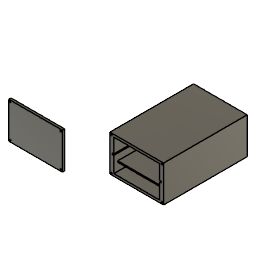
transmitter_model_v1 (Autodesk Fusion 360 design; units mm, degrees)
Autodesk Fusion 360 part; units mm, degrees
sketch "Sketch1" plane through (0, 0, 0) normal (0, 0, 1) x (1, 0, 0)
  line L0 (0, 0) -> (62, 0)
  line L1 (62, 0) -> (62, 82)
  line L2 (62, 82) -> (0, 82)
  line L3 (0, 82) -> (0, 0)
  dimension "d1" = 82
  dimension "d2" = 62
  constraint horizontal L0
  constraint vertical L1
  constraint horizontal L2
  constraint vertical L3
  constraint coincident L0.start L3.end
  measures "d1" distance of L0.start L2.end
  measures "d2" distance of L0.start L0.end
sketch "Sketch2" plane through (0, 0, 30) normal (0, 0, 1) x (-1, 0, 0)
  line L0 (0, -82) -> (0, 0)
  line L1 (0, 0) -> (-62, 0)
  line L2 (-62, 0) -> (-62, -82)
  line L3 (-62, -82) -> (0, -82)
  line L4 (-8, -8) -> (-54, -8)
  line L5 (-54, -8) -> (-54, -74)
  line L6 (-54, -74) -> (-8, -74)
  line L7 (-8, -74) -> (-8, -8)
  constraint horizontal L4
  constraint vertical L5
  constraint horizontal L6
  constraint vertical L7
sketch "Sketch3" plane through (0, 0, 0) normal (0, 0, 1) x (1, 0, 0)
  line L0 (0, 0) -> (62, 0)
  line L1 (62, 0) -> (62, 100)
  line L2 (62, 100) -> (0, 100)
  line L3 (0, 100) -> (0, 0)
  dimension "d11" = 100
  dimension "d12" = 62
  constraint horizontal L0
  constraint vertical L1
  constraint horizontal L2
  constraint vertical L3
  constraint coincident L0.start L3.end
  measures "d11" distance of L0.start L2.end
  measures "d12" distance of L0.start L0.end
extrude "Extrude3" add sketch "Sketch3" along normal blind 1.5 makes body 1
copy_body "CopyPasteBodies1" bodies 1 makes body 2
move_body "Move1" bodies 2 to x (1, 0, 0) y (0, 1, 0) z (0, 0, 1) at (-150, 0, 0)
extrude "Extrude4" add 1 faces at (62, 33.3333, 0.5) along direction (1, 0, 0) blind 8 on bodies 1 bodies 1
extrude "Extrude5" cut 1 faces at (70, 33.3333, 0.5) along direction (-1, 0, 0) blind 2 on bodies 1 bodies 1
extrude "Extrude6" add 1 faces at (45.3333, 100, 0.5) along direction (0, 1, 0) blind 6 on bodies 1 bodies 1
extrude "Extrude7" add 1 faces at (45.3333, 70.6667, 1.5) along direction (0, 0, 1) blind 44.5 on bodies 1 bodies 1
sketch "Sketch4" plane through (0, 0, 46) normal (0, 0, 1) x (-1, 0, 0)
  line L0 (-68, 0) -> (-68, -106)
  line L1 (-68, -106) -> (0, -106)
  line L2 (0, -106) -> (0, 0)
  line L3 (0, 0) -> (-68, 0)
  line L4 (0, 0) -> (-5, 0)
  line L5 (-68, 0) -> (-63, 0)
  line L6 (-5, 0) -> (-63, 0)
  line L7 (-63, 0) -> (-63, -101)
  line L8 (-63, -101) -> (-5, -101)
  line L9 (-5, -101) -> (-5, 0)
  dimension "d23" = 5
  dimension "d24" = 5
  dimension "d25" = 101
  dimension "d26" = 58
  constraint coincident L2.end L3.start
  constraint perpendicular L2 L4
  constraint coincident L0.start L3.end
  constraint perpendicular L0 L5
  constraint horizontal L6
  constraint vertical L7
  constraint horizontal L8
  constraint vertical L9
  measures "d23" distance of L2.end L4.end
  measures "d24" distance of L0.start L5.end
  measures "d25" distance of L4.end L8.end
  measures "d26" distance of L4.end L5.end
extrude "Extrude8" cut sketch "Sketch4" against normal blind 43 contours L3 L6 L7 L8 L9 bodies 1
extrude "Extrude9" add sketch "Sketch4" against normal blind 3 contours L3 L6 L7 L8 L9 bodies 1
move_body "Move2" bodies 2 to x (1, 0, 0) y (0, 1, 0) z (0, 0, 1) at (150, 0, -15)
move_body "Move3" bodies 2 to x (1, 0, 0) y (0, 1, 0) z (0, 0, 1) at (3, 0, 0)
copy_body "CopyPasteBodies2" bodies 2 makes body 3
move_body "Move4" bodies 3 to x (1, 0, 0) y (0, 1, 0) z (0, 0, 1) at (0, 0, 38)
move_body "Move5" bodies 3 to x (1, 0, 0) y (0, 1, 0) z (0, 0, 1) at (0, -100, 0)
extrude "Extrude11" add 1 faces at (23.6667, -100, 23.5) along direction (0, -1, 0) blind 3 on bodies 3 bodies 3
copy_body "CopyPasteBodies3" bodies 3 makes body 4
move_body "Move6" bodies 4 to x (1, 0, 0) y (0, 1, 0) z (0, 0, 1) at (0, 103, -10)
move_body "Move7" bodies 3 to x (1, 0, 0) y (0, 1, 0) z (0, 0, 1) at (0, 103, 0)
combine "Combine1" operation cut target body 1 tool bodies 3
combine "Combine2" operation add target body 1 tool bodies 4
sketch "Sketch5" plane through (0, 0, 0) normal (0, -1, 0) x (1, 0, 0)
  line L0 (63, 13) -> (63, 3)
  line L1 (63, 3) -> (5, 3)
  line L2 (5, 3) -> (5, 13)
  line L3 (5, 13) -> (63, 13)
  line L4 (68, 46) -> (0, 46)
  line L5 (0, 46) -> (0, 0)
  line L6 (0, 0) -> (68, 0)
  line L7 (68, 0) -> (68, 46)
  line L8 (63, 14.5) -> (5, 14.5)
  line L9 (5, 14.5) -> (5, 23)
  line L10 (5, 23) -> (3, 23)
  line L11 (3, 23) -> (3, 24.5)
  line L12 (3, 24.5) -> (5, 24.5)
  line L13 (5, 24.5) -> (5, 43)
  line L14 (5, 43) -> (63, 43)
  line L15 (63, 43) -> (63, 24.5)
  line L16 (63, 24.5) -> (65, 24.5)
  line L17 (65, 24.5) -> (65, 23)
  line L18 (65, 23) -> (63, 23)
  line L19 (63, 23) -> (63, 14.5)
  line L20 (5, 13) -> (63, 13)
  line L21 (63, 13) -> (63, 14.5)
  line L22 (63, 14.5) -> (5, 14.5)
  line L23 (5, 14.5) -> (5, 13)
  constraint horizontal L20
  constraint vertical L21
  constraint horizontal L22
  constraint vertical L23
  constraint coincident L8.start L19.end
  constraint coincident L2.end L3.start
extrude "Extrude12" cut sketch "Sketch5" against normal blind 5 contours L3 L8 L20 L21 L22 L23 bodies 1
move_body "Move8" bodies 2 1 to x (1, 0, 0) y (0, 1, 0) z (0, 0, 1) at (0, 25, 0)
sketch "Sketch6" plane through (0, 0, 0) normal (0, 1, 0) x (1, 0, 0)
  line L0 (0, 0) -> (68, 0)
  line L1 (68, 0) -> (68, -46)
  line L2 (68, -46) -> (0, -46)
  line L3 (0, -46) -> (0, 0)
  dimension "d37" = 46
  dimension "d38" = 68
  constraint horizontal L0
  constraint vertical L1
  constraint horizontal L2
  constraint vertical L3
  constraint coincident L0.start L3.end
  measures "d37" distance of L0.start L2.end
  measures "d38" distance of L1.end L2.end
extrude "Extrude13" add sketch "Sketch6" against normal blind 3 separate body makes body 5
move_body "Move9" bodies 5 to x (1, 0, 0) y (0, 1, 0) z (0, 0, 1) at (-100, 0, 0)
sketch "Sketch7" plane through (0, -3, 0) normal (0, -1, 0) x (1, 0, 0)
  line L0 (-32, 46) -> (-100, 46)
  line L1 (-100, 46) -> (-100, 0)
  line L2 (-100, 0) -> (-32, 0)
  line L3 (-32, 0) -> (-32, 46)
  line L4 (-100, 46) -> (-98, 46)
  line L5 (-98.3397, 46) -> (-98.3397, 44)
  circle A0 centre (-98.3397, 44) radius 1
  line L6 (-32, 46) -> (-34, 46)
  line L7 (-34, 46) -> (-34, 44)
  line L8 (-32, 0) -> (-32, 2)
  line L9 (-32, 2) -> (-34, 2)
  line L10 (-100, 0) -> (-100, 2)
  line L11 (-100, 2) -> (-98, 2)
  circle A1 centre (-34, 44) radius 1
  circle A2 centre (-34, 2) radius 1
  circle A3 centre (-98, 2) radius 1
  dimension "d41" = 2
  dimension "d42" = 2
  dimension "d43" = 2
  dimension "d44" = 2
  dimension "d45" = 2
  dimension "d46" = 2
  dimension "d47" = 2
  dimension "d48" = 2
  dimension "d49" = 2
  dimension "d50" = 2
  dimension "d51" = 2
  dimension "d52" = 2
  constraint coincident L0.end L1.start
  constraint perpendicular L1 L4
  constraint coincident L4 L5.start
  constraint perpendicular L4 L5
  constraint coincident L5.end A0.centre
  constraint coincident L0.start L3.end
  constraint perpendicular L3 L6
  constraint perpendicular L6 L7
  constraint coincident L2.end L3.start
  constraint perpendicular L2 L8
  constraint perpendicular L8 L9
  constraint coincident L1.end L2.start
  constraint perpendicular L2 L10
  constraint perpendicular L10 L11
  constraint coincident L7.end A1.centre
  constraint coincident L9.end A2.centre
  constraint coincident L11.end A3.centre
  measures "d41" distance of L0.end L4.end
  measures "d42" distance of L5.start L5.end
  measures "d43" diameter of A0
  measures "d44" distance of L0.start L6.end
  measures "d45" distance of L6.end L7.end
  measures "d46" distance of L2.end L8.end
  measures "d47" distance of L8.end L9.end
  measures "d48" distance of L1.end L10.end
  measures "d49" distance of L10.end L11.end
  measures "d50" diameter of A1
  measures "d51" diameter of A2
  measures "d52" diameter of A3
extrude "Extrude14" cut sketch "Sketch7" against normal blind 10 contours A0 | A1 | A2 | A3 bodies 5
sketch "Sketch8" plane through (0, 25, 0) normal (0, -1, 0) x (1, 0, 0)
  line L0 (5, 3) -> (5, 23)
  line L1 (5, 23) -> (3, 23)
  line L2 (3, 23) -> (3, 24.5)
  line L3 (3, 24.5) -> (5, 24.5)
  line L4 (5, 24.5) -> (5, 43)
  line L5 (5, 43) -> (63, 43)
  line L6 (63, 43) -> (63, 24.5)
  line L7 (63, 24.5) -> (65, 24.5)
  line L8 (65, 24.5) -> (65, 23)
  line L9 (65, 23) -> (63, 23)
  line L10 (63, 23) -> (63, 3)
  line L11 (63, 3) -> (5, 3)
  line L12 (68, 46) -> (0, 46)
  line L13 (0, 46) -> (0, 0)
  line L14 (0, 0) -> (68, 0)
  line L15 (68, 0) -> (68, 46)
  line L16 (0, 46) -> (2, 46)
  line L17 (2, 46) -> (2, 44)
  line L18 (0, 0) -> (0, 2)
  line L19 (0, 2) -> (2, 2)
  circle A0 centre (2, 2) radius 1
  line L20 (68, 0) -> (68, 2)
  line L21 (68, 2) -> (66, 2)
  circle A1 centre (66, 2) radius 1
  line L22 (68, 46) -> (66, 46)
  line L23 (66, 46) -> (66, 44)
  circle A2 centre (66, 44) radius 1
  circle A3 centre (2, 44) radius 1
  dimension "d55" = 2
  dimension "d56" = 2
  dimension "d57" = 2
  dimension "d58" = 2
  dimension "d59" = 2
  dimension "d60" = 2
  dimension "d61" = 2
  dimension "d62" = 2
  dimension "d63" = 2
  dimension "d64" = 2
  dimension "d65" = 2
  dimension "d66" = 2
  constraint coincident L12.end L13.start
  constraint perpendicular L13 L16
  constraint perpendicular L16 L17
  constraint coincident L13.end L14.start
  constraint perpendicular L14 L18
  constraint perpendicular L18 L19
  constraint coincident L19.end A0.centre
  constraint coincident L14.end L15.start
  constraint perpendicular L14 L20
  constraint perpendicular L20 L21
  constraint coincident L21.end A1.centre
  constraint coincident L12.start L15.end
  constraint perpendicular L15 L22
  constraint perpendicular L12 L23
  constraint coincident L23.end A2.centre
  constraint coincident L17.end A3.centre
  measures "d55" distance of L12.end L16.end
  measures "d56" distance of L16.end L17.end
  measures "d57" distance of L13.end L18.end
  measures "d58" distance of L18.end L19.end
  measures "d59" diameter of A0
  measures "d60" distance of L14.end L20.end
  measures "d61" distance of L20.end L21.end
  measures "d62" diameter of A1
  measures "d63" distance of L12.start L22.end
  measures "d64" distance of L22.end L23.end
  measures "d65" diameter of A2
  measures "d66" diameter of A3
extrude "Extrude15" cut sketch "Sketch8" against normal blind 10 contours A0 | A1 | A2 | A3 bodies 1
extrude "Extrude10" [rolled back] along distance 3 taper angle 0
hidden bodies 2
